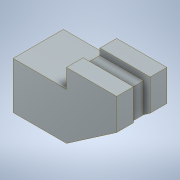
# Autodesk Inventor part: under walle L3
Saved by Autodesk Inventor 2022 (Build 260153000, 153)
## iProperties
Created: 2021-12-22
Part Number: under walle L3
Material: Generic
Document SubType Name: Modeling
Designer: MatusBarany
Density: 1 g/cm^3
Appearance: Foil Gold
Author: MatusBarany
Autodesk Inventor part; units mm, degrees
ref_plane "YZ Plane" through (0, 0, 0) normal (1, 0, 0) x (0, 1, 0)
ref_plane "XZ Plane" through (0, 0, 0) normal (0, 1, 0) x (-1, 0, 0)
ref_plane "XY Plane" through (0, 0, 0) normal (0, 0, 1) x (1, 0, 0)
sketch "Sketch1" plane through (0, 0, 0) normal (0, 0, 1) x (1, 0, 0)
  line L0 (-30.7315, 6.2426) -> (-13.7315, 6.2426)
  line L1 (-13.7315, 6.2426) -> (-13.7315, -8.7574)
  line L2 (-13.7315, -8.7574) -> (-30.7315, -8.7574)
  line L3 (-30.7315, -8.7574) -> (-30.7315, 6.2426)
  line L4 (2.2685, 2.2426) -> (2.2685, 12.2426)
  line L5 (2.2685, 12.2426) -> (-13.7315, 12.2426)
  line L6 (-13.7315, 12.2426) -> (-13.7315, 6.2426)
  line L7 (-13.7315, -8.7574) -> (2.2685, 2.2426)
  point P0 (0, 0)
  dimension "d0" = 15
  dimension "d1" = 17
  dimension "d2" = 6
  dimension "d3" = 16
  dimension "d4" = 10
  constraints: 16 end point, 3 parallel, 2 perpendicular, 1 horizontal
  measures "d0" distance of L2.end L0.start
  measures "d1" distance of L0.start L0.end
  measures "d2" distance of L5.end L0.end
  measures "d3" distance of L4.end L5.end
  measures "d4" distance of L4.start L4.end
extrude "Extrusion1" add sketch "Sketch1" along normal blind 16
sketch "Sketch2" plane through (-13.7315, 12.2426, 0) normal (0, 1, 0) x (1, 0, 0)
  line L0 (16, 0) -> (16, -16) projected
  line L1 (0, -5.3333) -> (16, -5.3333)
  line L2 (16, -5.3333) -> (16, -10.6667)
  line L3 (16, -10.6667) -> (0, -10.6667)
  line L4 (0, -10.6667) -> (0, -5.3333)
  line L5 (0, 0) -> (0, -16) projected
  line L6 (16, 0) -> (0, 0) projected
  line L7 (16, -16) -> (0, -16) projected
  point P0 (13.7315, 0)
  dimension "d7" = 16
  dimension "d8" = 5.3333
  dimension "d9" = 5.3333
  constraints: 8 end point, 2 parallel, 2 point on line, 1 horizontal, 1 perpendicular
  measures "d7" distance of L0.start L0.end
  measures "d8" distance between parallel lines of L3 L1
  measures "d9" distance between parallel lines of L6 L1
extrude "Extrusion2" cut sketch "Sketch2" against normal blind 2 contours L0 L3 L4 L1
sketch "Sketch3" plane through (2.2685, 2.2426, 0) normal (1, 0, 0) x (0, 0, -1)
  line L0 (-10.6667, 8) -> (-10.6667, 10) projected
  line L1 (-10.6667, 10) -> (-16, 10) projected
  line L2 (-16, 0) -> (-16, 10) projected
  line L3 (0, 0) -> (-16, 0) projected
  line L4 (0, 0) -> (0, 10) projected
  line L5 (0, 10) -> (-5.3333, 10) projected
  line L6 (-5.3333, 10) -> (-5.3333, 8) projected
  line L7 (-5.3333, 8) -> (-10.6667, 8) projected
  line L8 (0, 0) -> (-16, 0) projected
  line L9 (-10.6667, 8) -> (-5.3333, 8)
  line L10 (-10.6667, 8) -> (-10.6667, -2)
  line L11 (-10.6667, -2) -> (-5.3333, -2)
  line L12 (-5.3333, -2) -> (-5.3333, 8)
  point P0 (0, -2.2426)
  dimension "d14" = 10
  dimension "d15" = 10
  constraints: 8 end point, 1 horizontal, 1 parallel, 1 perpendicular, 1 vertical
  measures "d14" distance of L11.end L6.end
  measures "d15" distance of L3.start L4.end
extrude "Extrusion3" cut sketch "Sketch3" against normal blind 2 contours L7 L12 L3 L10 | L3 L12 L11 L10
sketch "Sketch4" plane through (-13.7315, -8.7574, 0) normal (0.5665288, -0.8240419, 0) x (0.8240419, 0.5665288, 0)
  line L0 (16.9894, 10.6667) -> (19.4165, 10.6667) projected
  line L1 (19.4165, 10.6667) -> (19.4165, 16) projected
  line L2 (0, 16) -> (19.4165, 16) projected
  line L3 (0, 0) -> (0, 16) projected
  line L4 (0, 0) -> (19.4165, 0) projected
  line L5 (19.4165, 0) -> (19.4165, 5.3333) projected
  line L6 (19.4165, 5.3333) -> (16.9894, 5.3333) projected
  line L7 (16.9894, 5.3333) -> (16.9894, 10.6667) projected
  line L8 (16.9894, 10.6667) -> (19.4165, 10.6667) projected
  line L9 (16.9894, 10.6667) -> (0, 10.6667)
  line L10 (0, 10.6667) -> (0, 5.3333)
  line L11 (0, 5.3333) -> (16.9894, 5.3333)
  line L12 (16.9894, 5.3333) -> (16.9894, 10.6667)
  point P0 (16.2766, 0)
  dimension "d17" = 19.4165
  constraints: 8 end point, 2 parallel, 1 horizontal, 1 perpendicular, 1 point on line
  measures "d17" distance of L3.start L4.end
extrude "Extrusion4" cut sketch "Sketch4" against normal blind 2 contours L7 L11 L3 L9
chamfer "Chamfer1" distance 2 angle 45 1 edges at (-14.8657, -7.1076, 8)
sketch "Sketch5" plane through (-30.7315, -8.7574, 0) normal (-1, 0, 0) x (0, 0, 1)
  line L0 (6, 13) -> (10, 13)
  line L1 (10, 13) -> (10, 2)
  line L2 (10, 2) -> (6, 2)
  line L3 (6, 2) -> (6, 13)
  line L4 (0, 15) -> (0, 0) projected
  line L5 (0, 0) -> (16, 0) projected
  line L6 (16, 15) -> (16, 0) projected
  line L7 (0, 15) -> (16, 15) projected
  point P0 (0, 8.7574)
  dimension "d23" = 4
  dimension "d24" = 11
  dimension "d25" = 6
  dimension "d26" = 15
  dimension "d27" = 16
  dimension "d28" = 2
  constraints: 8 end point, 2 parallel, 1 horizontal, 1 perpendicular
  measures "d23" distance of L0.start L0.end
  measures "d24" distance of L0.end L1.end
  measures "d25" distance between parallel lines of L6 L1
  measures "d26" distance of L6.start L5.end
  measures "d27" distance of L4.start L6.start
  measures "d28" distance between parallel lines of L7 L0
extrude "Extrusion5" cut sketch "Sketch5" against normal blind 5 contours L0 L1 L2 L3
equation "\"d8\" = 0.333333 * d7"
equation "\"d9\" = -2 * d8 + d7"
equation "\"d14\" = d15"
equation "\"d25\" = -0.5 * d23 + 0.5 * d27"
equation "\"d28\" = -0.5 * d24 + 0.5 * d26"
body "Solid1"
